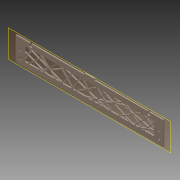
# Autodesk Inventor part: Panel_front
Saved by Autodesk Inventor 2013 (Build 170138000, 138)
## iProperties
Created: 2013-02-02
Part Number: Panel_front
Material: Aluminum 6061
Document SubType Name: Modeling
Designer: xylzlyx
Density: 1 g/cm^3
Author: xylzlyx
Autodesk Inventor part; units mm, degrees
ref_plane "YZ Plane" through (0, 0, 0) normal (1, 0, 0) x (0, 1, 0)
ref_plane "XZ Plane" through (0, 0, 0) normal (0, 1, 0) x (-1, 0, 0)
ref_plane "XY Plane" through (0, 0, 0) normal (0, 0, 1) x (1, 0, 0)
ref_plane "Work Plane1" through (0, 0, -9.525) normal (0, 0, 1) x (1, 0, 0)
sketch "Sketch1" plane through (0, 0, -9.525) normal (0, 0, 1) x (1, 0, 0)
  line L0 (381, -60.8043) -> (381, -64.0283) construction
  line L1 (381, -64.0283) -> (0, -64.0283) construction
  line L2 (0, -64.0283) -> (0, -60.8043) construction
  line L3 (0, -60.8043) -> (381, -60.8043) construction
  line L4 (381, 0) -> (0, 0) construction
  line L5 (0, 0) -> (0, 3.175) construction
  line L6 (0, 3.175) -> (381, 3.175) construction
  line L7 (381, 3.175) -> (381, 0) construction
  line L8 (381, -60.8043) -> (0, -60.8043)
  line L9 (0, -60.8043) -> (0, 0)
  line L10 (0, 0) -> (381, 0)
  line L11 (381, 0) -> (381, -60.8043)
  constraints: 24 end point, 5 horizontal, 4 coincident, 4 vertical, 2 parallel, 1 perpendicular, 8 other
extrude "FrontPanel" add sketch "Sketch1" against normal blind 3.175
fillet "CornerFillet" radius 1 4 edges at (381, -60.8043, -11.1125) (0, -60.8043, -11.1125) (0, 0, -11.1125) (381, 0, -11.1125)
sketch "ScrewSlotSketch" plane through (0, 0, -9.525) normal (0, 0, 1) x (1, 0, 0)
  line L0 (368.3, -28.0035) -> (368.3, -1) projected
  line L1 (12.7, -1) -> (12.7, -28.0035) projected
  line L2 (381, 0) -> (0, 0) construction
  line L3 (0, 0) -> (0, 3.175) construction
  line L4 (0, 3.175) -> (381, 3.175) construction
  line L5 (381, 3.175) -> (381, 0) construction
  line L6 (381, -60.8043) -> (381, -64.0283) construction
  line L7 (381, -64.0283) -> (0, -64.0283) construction
  line L8 (0, -64.0283) -> (0, -60.8043) construction
  line L9 (0, -60.8043) -> (381, -60.8043) construction
  line L10 (344.7987, -8.89) -> (344.7987, 3.175)
  line L11 (344.7987, 3.175) -> (341.0014, 3.175)
  line L12 (341.0014, 3.175) -> (341.0014, -8.89)
  line L13 (341.0014, -8.89) -> (344.7987, -8.89)
  line L14 (346.9958, -8.89) -> (338.8043, -8.89)
  line L15 (338.8043, -8.89) -> (338.8043, -5.8579)
  line L16 (338.8043, -5.8579) -> (346.9958, -5.8579)
  line L17 (346.9958, -5.8579) -> (346.9958, -8.89)
  line L18 (36.2014, -8.89) -> (39.9987, -8.89)
  line L19 (39.9987, -8.89) -> (39.9987, 3.175)
  line L20 (39.9987, 3.175) -> (36.2014, 3.175)
  line L21 (36.2014, 3.175) -> (36.2014, -8.89)
  line L22 (34.0043, -8.89) -> (42.1958, -8.89)
  line L23 (42.1958, -8.89) -> (42.1958, -5.8579)
  line L24 (42.1958, -5.8579) -> (34.0043, -5.8579)
  line L25 (34.0043, -5.8579) -> (34.0043, -8.89)
  point P0 (342.9, 3.175)
  point P1 (342.9, -8.89)
  point P2 (38.1, -8.89)
  point P3 (38.1, 3.175)
  dimension "d4" = 12.065
  dimension "d6" = 3.7973
  dimension "d7" = 25.4
  dimension "d8" = 8.1915
  dimension "d9" = 3.0321
  dimension "d10" = 3.7973
  dimension "d11" = 12.065
  dimension "d12" = 8.1915
  dimension "d13" = 3.0321
  dimension "d14" = 25.4
  constraints: 48 end point, 11 parallel, 6 horizontal, 6 midpoint, 4 vertical, 2 perpendicular, 2 point on line, 1 collinear, 7 other
  measures "d4" distance of L10.start L10.end
  measures "d6" distance of L10.end L11.end
  measures "d7" distance from line of L0 point (342.9, 3.175)
  measures "d8" distance of L14.start L14.end
  measures "d9" distance of L14.end L15.end
  measures "d10" distance of L19.end L20.end
  measures "d11" distance of L20.end L18.start
  measures "d12" distance of L22.start L22.end
  measures "d13" distance of L22.end L23.end
  measures "d14" distance from line of L1 point (38.1, 3.175)
extrude "ScrewSlotExtrusion" cut sketch "ScrewSlotSketch" against normal blind 3.175
fillet "ScrewSlotFillet" radius 0.5 16 edges at (344.7987, 0, -11.1125) (341.0014, 0, -11.1125) (344.7987, -5.8579, -11.1125) (341.0014, -5.8579, -11.1125) (338.8043, -5.8579, -11.1125) (338.8043, -8.89, -11.1125) (346.9958, -8.89, -11.1125) (346.9958, -5.8579, -11.1125) (42.1958, -8.89, -11.1125) (42.1958, -5.8579, -11.1125) (39.9987, -5.8579, -11.1125) (39.9987, 0, -11.1125) (36.2014, 0, -11.1125) (36.2014, -5.8579, -11.1125) (34.0043, -5.8579, -11.1125) (34.0043, -8.89, -11.1125)
sketch "ScrewHoleSketch" plane through (0, 0, -9.525) normal (0, 0, 1) x (1, 0, 0)
  line L0 (34.0043, -8.39) -> (34.0043, -6.3579) projected
  line L1 (368.3, -28.5035) -> (371.475, -28.5035) projected
  line L2 (371.475, -32.3008) -> (368.3, -32.3008) projected
  line L3 (9.525, -28.5035) -> (12.7, -28.5035) projected
  line L4 (12.7, -32.3008) -> (9.525, -32.3008) projected
  line L5 (371.475, -28.5035) -> (371.475, -32.3008) construction
  line L6 (9.525, -28.5035) -> (9.525, -32.3008) construction
  point P0 (0, 0)
  point P1 (11.1125, -30.4021)
  point P2 (369.8875, -30.4021)
  point P3 (369.8875, -28.5035)
  point P4 (371.475, -30.4021)
  point P5 (9.525, -30.4021)
  point P6 (11.1125, -28.5035)
  constraints: 4 end point, 4 midpoint, 2 horizontal alignment, 2 parallel, 2 vertical alignment
hole "ScrewHoles" at (11.1125, -30.4021, -9.525) at (369.8875, -30.4021, -9.525) direction (0, 0, -1) diameter 3.7973 end through all
sketch "BottomTabSketch" plane through (40.4987, 0, -9.525) normal (0, 1, 0) x (1, 0, 0)
  line L0 (162.7014, 3.175) -> (137.3014, 3.175)
  line L1 (137.3014, 3.175) -> (137.3014, 0)
  line L2 (137.3014, 0) -> (162.7014, 0)
  line L3 (162.7014, 0) -> (162.7014, 3.175)
  line L4 (137.0473, 2.929) -> (137.0473, 0.246) projected
  line L5 (137.5473, -0.254) -> (162.4553, -0.254) projected
  point P0 (0, 3.175)
  point P1 (-40.4987, -9.525)
  point P2 (137.3014, 1.5875)
  point P3 (137.0473, 1.5875)
  point P4 (150.0014, 0)
  point P5 (150.0013, -0.254)
  dimension "d29" = 25.4
  constraints: 8 end point, 4 midpoint, 2 horizontal alignment, 2 parallel, 1 horizontal, 1 perpendicular, 1 vertical alignment
  measures "d29" distance of L0.start L0.end
extrude "BottomTab" add sketch "BottomTabSketch" along normal blind 3.175
fillet "BottomTabFillet" radius 0.5 4 edges at (177.8, 0, -11.1125) (177.8, 3.175, -11.1125) (203.2, 3.175, -11.1125) (203.2, 0, -11.1125)
sketch "SlotSketch" plane through (0, 0, -9.525) normal (0, 0, 1) x (1, 0, 0)
  circle A0 centre (11.1125, -30.4021) radius 1.8986 projected
  circle A1 centre (369.8875, -30.4021) radius 1.8986 projected
  line L0 (371.729, -50.6197) -> (368.046, -50.6197)
  line L1 (368.046, -50.6197) -> (368.046, -40.5867)
  line L2 (368.046, -40.5867) -> (371.729, -40.5867)
  line L3 (371.729, -40.5867) -> (371.729, -50.6197)
  line L4 (12.954, -50.6197) -> (9.271, -50.6197)
  line L5 (9.271, -50.6197) -> (9.271, -40.5867)
  line L6 (9.271, -40.5867) -> (12.954, -40.5867)
  line L7 (12.954, -40.5867) -> (12.954, -50.6197)
  line L8 (380, -60.8043) -> (1, -60.8043) projected
  line L9 (203.2, 0.5) -> (203.2, 2.675) projected
  line L10 (11.1125, -30.4021) -> (11.1125, -60.8043) construction
  line L11 (369.8875, -30.4021) -> (369.8875, -60.8043) construction
  point P0 (0, 0)
  point P1 (12.954, -45.6032)
  point P2 (11.1125, -45.6032)
  point P3 (11.1125, -50.6197)
  point P4 (369.8875, -45.6032)
  point P5 (371.729, -45.6032)
  point P6 (369.8875, -50.6197)
  dimension "d34" = 10.033
  dimension "d36" = 3.683
  dimension "d37" = 10.033
  dimension "d38" = 3.683
  constraints: 20 end point, 6 midpoint, 6 parallel, 2 horizontal, 2 horizontal alignment, 2 perpendicular, 2 point on line, 2 vertical alignment
  measures "d34" distance of L0.end L1.end
  measures "d36" distance of L0.start L0.end
  measures "d37" distance of L6.end L4.start
  measures "d38" distance of L4.start L4.end
extrude "Extrusion4" cut sketch "SlotSketch" against normal blind 3.175 contours L0 L1 L2 L3 | L4 L5 L6 L7
fillet "Fillet5" radius 0.5 8 edges at (368.046, -40.5867, -11.1125) (371.729, -40.5867, -11.1125) (371.729, -50.6197, -11.1125) (368.046, -50.6197, -11.1125) (9.271, -40.5867, -11.1125) (12.954, -40.5867, -11.1125) (12.954, -50.6197, -11.1125) (9.271, -50.6197, -11.1125)
sketch "Sketch6" plane through (0, 0, -9.525) normal (0, 0, 1) x (1, 0, 0)
  line L0 (380, -60.8043) -> (1, -60.8043) projected
  line L1 (203.7, 0) -> (340.5014, 0) projected
  circle A0 centre (11.1125, -30.4021) radius 1.8986 projected
  circle A1 centre (369.8875, -30.4021) radius 1.8986 projected
  line L2 (357.1875, -48.1043) -> (23.8125, -48.1043)
  line L3 (23.8125, -48.1043) -> (23.8125, -12.7)
  line L4 (23.8125, -12.7) -> (357.1875, -12.7)
  line L5 (357.1875, -12.7) -> (357.1875, -48.1043)
  point P0 (0, 0)
  dimension "d42" = 12.7
  dimension "d43" = 12.7
  dimension "d44" = 12.7
  dimension "d45" = 12.7
  constraints: 8 end point, 2 parallel, 1 horizontal, 1 perpendicular
  measures "d42" distance from line of L0 L2.start
  measures "d43" distance between parallel lines of L1 L4
  measures "d44" distance from line of A1.centre L5
  measures "d45" distance from line of A0.centre L3
extrude "Extrusion5" cut sketch "Sketch6" against normal blind 25.4 contours L2 L3 L4 L5
fillet "Fillet6" radius 0.5 4 edges at (357.1875, -48.1043, -11.1125) (357.1875, -12.7, -11.1125) (23.8125, -48.1043, -11.1125) (23.8125, -12.7, -11.1125)
sketch "Sketch7" plane through (0, 0, -9.525) normal (0, 0, 1) x (1, 0, 0)
  line L0 (357.1875, -13.2) -> (357.1875, -47.6043) projected
  line L1 (356.6875, -48.1043) -> (24.3125, -48.1043) projected
  line L2 (23.8125, -47.6043) -> (23.8125, -13.2) projected
  line L3 (24.3125, -12.7) -> (356.6875, -12.7) projected
  arc A0 (357.1875, -13.2) -> (356.6875, -12.7) centre (356.6875, -13.2) ccw projected
  line L4 (203.7, 0) -> (340.5014, 0) projected
  line L5 (357.1875, -36.7105) -> (321.9415, -48.1043)
  line L6 (357.1875, -21.5969) -> (332.397, -48.1043)
  line L7 (344.6458, -12.7) -> (309.178, -48.1043)
  line L8 (326.9119, -12.7) -> (268.5984, -48.1043)
  line L9 (304.4629, -12.7) -> (185.3162, -48.1043)
  line L10 (278.4902, -12.7) -> (215.3456, -48.1043)
  line L11 (237.5513, -12.7) -> (203.2, -48.1043)
  line L12 (212.9458, -12.7) -> (157.4642, -48.1043)
  line L13 (168.7522, -12.7) -> (144.5905, -48.1043)
  line L14 (147.217, -12.7) -> (120.8379, -48.1043)
  line L15 (131.8636, -12.7) -> (62.8918, -48.1043)
  line L16 (105.8433, -12.7) -> (72.2367, -48.1043)
  line L17 (74.5284, -12.7) -> (34.5043, -48.1043)
  line L18 (41.1958, -12.7) -> (23.8125, -42.1574)
  line L19 (357.1875, -36.7105) -> (357.1875, -34.575)
  line L20 (357.1875, -34.575) -> (315.3354, -48.1043)
  line L21 (321.9415, -48.1043) -> (315.3354, -48.1043)
  line L22 (357.1875, -21.5969) -> (357.1875, -18.622)
  line L23 (357.1875, -18.622) -> (329.6149, -48.1043)
  line L24 (329.6149, -48.1043) -> (332.397, -48.1043)
  line L25 (344.6458, -12.7) -> (341.7696, -12.7)
  line L26 (341.7696, -12.7) -> (306.3017, -48.1043)
  line L27 (309.178, -48.1043) -> (306.3017, -48.1043)
  line L28 (326.9119, -12.7) -> (322.9965, -12.7)
  line L29 (322.9965, -12.7) -> (264.683, -48.1043)
  line L30 (264.683, -48.1043) -> (268.5984, -48.1043)
  line L31 (304.4629, -12.7) -> (297.3291, -12.7)
  line L32 (297.3291, -12.7) -> (178.1824, -48.1043)
  line L33 (185.3162, -48.1043) -> (178.1824, -48.1043)
  line L34 (278.4902, -12.7) -> (274.3353, -12.7)
  line L35 (274.3353, -12.7) -> (211.1907, -48.1043)
  line L36 (208.3319, -48.1043) -> (215.3456, -48.1043)
  line L37 (237.5513, -12.7) -> (234.72, -12.7)
  line L38 (234.72, -12.7) -> (200.3687, -48.1043)
  line L39 (203.2, -48.1043) -> (200.3687, -48.1043)
  line L40 (212.9458, -12.7) -> (209.1683, -12.7)
  line L41 (209.1683, -12.7) -> (153.6867, -48.1043)
  line L42 (157.4642, -48.1043) -> (153.6867, -48.1043)
  line L43 (168.7522, -12.7) -> (166.2921, -12.7)
  line L44 (166.2921, -12.7) -> (142.1304, -48.1043)
  line L45 (142.1304, -48.1043) -> (144.5905, -48.1043)
  line L46 (147.217, -12.7) -> (144.683, -12.7)
  line L47 (144.683, -12.7) -> (118.3039, -48.1043)
  line L48 (120.8379, -48.1043) -> (118.3039, -48.1043)
  line L49 (131.8636, -12.7) -> (127.4139, -12.7)
  line L50 (127.4139, -12.7) -> (58.4422, -48.1043)
  line L51 (58.4422, -48.1043) -> (62.8918, -48.1043)
  line L52 (105.8433, -12.7) -> (103.0416, -12.7)
  line L53 (103.0416, -12.7) -> (69.4351, -48.1043)
  line L54 (69.4351, -48.1043) -> (72.2367, -48.1043)
  line L55 (74.5284, -12.7) -> (71.4615, -12.7)
  line L56 (71.4615, -12.7) -> (31.4373, -48.1043)
  line L57 (34.5043, -48.1043) -> (31.4373, -48.1043)
  line L58 (41.1958, -12.7) -> (38.8363, -12.7)
  line L59 (38.8363, -12.7) -> (23.8125, -38.1592)
  line L60 (23.8125, -42.1574) -> (23.8125, -38.1592)
  point P0 (0, 0)
  dimension "d49" = 23.5105
  dimension "d50" = 8.3969
  dimension "d51" = 72.086
  dimension "d52" = 43.083
  dimension "d53" = 12.0417
  dimension "d54" = 29.7756
  dimension "d55" = 135.051
  dimension "d56" = 148.736
  dimension "d57" = 52.2246
  dimension "d58" = 163.451
  dimension "d59" = 78.1973
  dimension "d60" = 150.721
  dimension "d61" = 119.1362
  dimension "d62" = 134.135
  dimension "d63" = 143.7417
  dimension "d64" = 147.457
  dimension "d65" = 187.9353
  dimension "d66" = 124.312
  dimension "d67" = 209.4705
  dimension "d68" = 126.689
  dimension "d69" = 224.8239
  dimension "d70" = 152.828
  dimension "d71" = 250.8442
  dimension "d72" = 133.508
  dimension "d73" = 282.1591
  dimension "d74" = 138.505
  dimension "d75" = 315.4918
  dimension "d76" = 120.545
  dimension "d77" = 2.032
  dimension "d78" = 2.032
  dimension "d79" = 2.032
  dimension "d80" = 2.032
  dimension "d81" = 2.032
  dimension "d82" = 2.032
  dimension "d83" = 2.032
  dimension "d84" = 2.032
  dimension "d85" = 2.032
  dimension "d86" = 2.032
  dimension "d87" = 2.032
  dimension "d88" = 2.032
  dimension "d89" = 2.032
  dimension "d90" = 2.032
  constraints: 112 end point, 16 parallel, 10 horizontal, 6 point on line, 1 collinear, 53 other
  measures "d49" vertical distance of A0.centre L5.start
  measures "d50" vertical distance of A0.centre L6.start
  measures "d51" angle of L0 L5
  measures "d52" angle of L0 L6
  measures "d53" distance of A0.end L7.start
  measures "d54" distance of A0.end L8.start
  measures "d55" angle to the sketch x axis of L7
  measures "d56" angle to the sketch x axis of L8
  measures "d57" distance of A0.end L9.start
  measures "d58" angle to the sketch x axis of L9
  measures "d59" distance of A0.end L10.start
  measures "d60" angle to the sketch x axis of L10
  measures "d61" distance of A0.end L11.start
  measures "d62" angle to the sketch x axis of L11
  measures "d63" distance of A0.end L12.start
  measures "d64" angle to the sketch x axis of L12
  measures "d65" distance of A0.end L13.start
  measures "d66" angle to the sketch x axis of L13
  measures "d67" distance of A0.end L14.start
  measures "d68" angle to the sketch x axis of L14
  measures "d69" distance of A0.end L15.start
  measures "d70" angle to the sketch x axis of L15
  measures "d71" distance of A0.end L16.start
  measures "d72" angle to the sketch x axis of L16
  measures "d73" distance of A0.centre L17.start
  measures "d74" angle to the sketch x axis of L17
  measures "d75" distance of A0.centre L18.start
  measures "d76" angle to the sketch x axis of L18
  measures "d77" distance between parallel lines of L5 L20
  measures "d78" distance between parallel lines of L6 L23
  measures "d79" distance between parallel lines of L7 L26
  measures "d80" distance between parallel lines of L8 L29
  measures "d81" distance between parallel lines of L9 L32
  measures "d82" distance between parallel lines of L10 L35
  measures "d83" distance between parallel lines of L38 L11
  measures "d84" distance between parallel lines of L41 L12
  measures "d85" distance between parallel lines of L44 L13
  measures "d86" distance between parallel lines of L14 L47
  measures "d87" distance between parallel lines of L15 L50
  measures "d88" distance between parallel lines of L16 L53
  measures "d89" distance between parallel lines of L17 L56
  measures "d90" distance between parallel lines of L18 L59
extrude "Hash1" add sketch "Sketch7" against normal blind 3.175 contours L0 L6 L20 L23 | L23 L5 L1 L20 | L20 L6 L5 L23 | L7 L1 L26 L3 | L0 L5 L6 L20 | L5 L6 L1 L23 | L8 L1 L29 L3 | L9 L10 L32 L3 | L10 L1 L35 L9 | L9 L35 L32 L10 | L10 L32 L35 L3 | L9 L11 L32 L35 | L11 L1 L38 L9 | L9 L38 L32 L11 | L11 L32 L38 L3 | L9 L1 L32 L38 | L12 L1 L41 L3 | L13 L1 L44 L3 | L14 L1 L47 L3 | L15 L16 L50 L3 | L16 L1 L53 L15 | L15 L53 L50 L16 | L16 L50 L53 L3 | L15 L1 L50 L53 | L17 L1 L56 L3 | L2 L59 L3 L18
sketch "Sketch8" plane through (0, 0, -9.525) normal (0, 0, 1) x (1, 0, 0)
  line L0 (212.9458, -12.7) -> (234.72, -12.7) projected
  line L1 (304.4629, -12.7) -> (322.9965, -12.7) projected
  line L2 (264.683, -48.1043) -> (215.3456, -48.1043) projected
  line L3 (200.3687, -48.1043) -> (185.3162, -48.1043) projected
  line L4 (237.5513, -12.7) -> (274.3353, -12.7) projected
  line L5 (118.3039, -48.1043) -> (72.2367, -48.1043) projected
  line L6 (74.5284, -12.7) -> (103.0416, -12.7) projected
  line L7 (357.1875, -36.7105) -> (357.1875, -47.6043) projected
  arc A0 (357.1875, -13.2) -> (356.6875, -12.7) centre (356.6875, -13.2) ccw projected
  line L8 (329.6149, -48.1043) -> (321.9415, -48.1043) projected
  line L9 (153.6867, -48.1043) -> (144.5905, -48.1043) projected
  line L10 (168.7522, -12.7) -> (209.1683, -12.7) projected
  line L11 (306.3017, -48.1043) -> (268.5984, -48.1043) projected
  line L12 (326.9119, -12.7) -> (341.7696, -12.7) projected
  line L13 (147.217, -12.7) -> (166.2921, -12.7) projected
  line L14 (23.8125, -38.1592) -> (23.8125, -13.2) projected
  line L15 (24.3125, -12.7) -> (38.8363, -12.7) projected
  line L16 (105.8433, -12.7) -> (127.4139, -12.7) projected
  line L17 (41.1958, -12.7) -> (71.4615, -12.7) projected
  line L18 (278.4902, -12.7) -> (297.3291, -12.7) projected
  line L19 (357.1875, -21.5969) -> (357.1875, -34.575) projected
  line L20 (243.5183, -12.7) -> (357.1875, -39.9851)
  line L21 (279.4501, -12.7) -> (324.0356, -48.1043)
  line L22 (206.4666, -12.7) -> (243.5183, -48.1043)
  line L23 (171.4741, -12.7) -> (198.865, -48.1043)
  line L24 (120.8379, -12.7) -> (227.4264, -48.1043)
  line L25 (112.4755, -12.7) -> (146.4133, -48.1043)
  line L26 (328.1908, -12.7) -> (357.1875, -33.5005)
  line L27 (219.5665, -12.7) -> (293.0889, -48.1043)
  line L28 (60.7242, -12.7) -> (101.1114, -48.1043)
  line L29 (29.3613, -12.7) -> (116.1142, -48.1043)
  line L30 (23.8125, -28.5035) -> (75.6529, -48.1043)
  line L31 (328.1908, -12.7) -> (331.677, -12.7)
  line L32 (331.677, -12.7) -> (357.1875, -30.9997)
  line L33 (357.1875, -33.5005) -> (357.1875, -30.9997)
  line L34 (279.4501, -12.7) -> (282.7177, -12.7)
  line L35 (282.7177, -12.7) -> (327.3032, -48.1043)
  line L36 (327.3032, -48.1043) -> (324.0356, -48.1043)
  line L37 (243.5183, -12.7) -> (252.224, -12.7)
  line L38 (252.224, -12.7) -> (357.1875, -37.8954)
  line L39 (357.1875, -37.8954) -> (357.1875, -39.9851)
  line L40 (219.5665, -12.7) -> (224.25, -12.7)
  line L41 (224.25, -12.7) -> (297.7725, -48.1043)
  line L42 (297.7725, -48.1043) -> (293.0889, -48.1043)
  line L43 (243.5183, -48.1043) -> (246.4596, -48.1043)
  line L44 (246.4596, -48.1043) -> (209.4079, -12.7)
  line L45 (209.4079, -12.7) -> (206.4666, -12.7)
  line L46 (227.4264, -48.1043) -> (233.8726, -48.1043)
  line L47 (233.8726, -48.1043) -> (127.2841, -12.7)
  line L48 (120.8379, -12.7) -> (127.2841, -12.7)
  line L49 (146.4133, -48.1043) -> (149.2281, -48.1043)
  line L50 (149.2281, -48.1043) -> (115.2903, -12.7)
  line L51 (115.2903, -12.7) -> (112.4755, -12.7)
  line L52 (116.1142, -48.1043) -> (121.492, -48.1043)
  line L53 (121.492, -48.1043) -> (34.7391, -12.7)
  line L54 (34.7391, -12.7) -> (29.3613, -12.7)
  line L55 (60.7242, -12.7) -> (63.8068, -12.7)
  line L56 (63.8068, -12.7) -> (104.194, -48.1043)
  line L57 (101.1114, -48.1043) -> (104.194, -48.1043)
  line L58 (75.6529, -48.1043) -> (81.3985, -48.1043)
  line L59 (81.3985, -48.1043) -> (23.8125, -26.3311)
  line L60 (23.8125, -26.3311) -> (23.8125, -28.5035)
  line L61 (198.865, -48.1043) -> (201.4341, -48.1043)
  line L62 (201.4341, -48.1043) -> (174.0432, -12.7)
  line L63 (174.0432, -12.7) -> (171.4741, -12.7)
  point P0 (0, 0)
  dimension "d93" = 28.4967
  dimension "d94" = 77.2374
  dimension "d95" = 113.1692
  dimension "d96" = 137.121
  dimension "d97" = 150.2209
  dimension "d98" = 185.2134
  dimension "d99" = 235.8496
  dimension "d100" = 244.212
  dimension "d101" = 295.9633
  dimension "d102" = 327.3262
  dimension "d103" = 15.3035
  dimension "d104" = 144.347
  dimension "d105" = 141.548
  dimension "d106" = 166.502
  dimension "d107" = 154.287
  dimension "d108" = 136.302
  dimension "d109" = 127.728
  dimension "d110" = 161.626
  dimension "d111" = 133.788
  dimension "d112" = 138.762
  dimension "d113" = 157.799
  dimension "d114" = 69.288
  dimension "d115" = 2.032
  dimension "d116" = 2.032
  dimension "d117" = 2.032
  dimension "d118" = 2.032
  dimension "d119" = 2.032
  dimension "d120" = 2.032
  dimension "d121" = 2.032
  dimension "d122" = 2.032
  dimension "d123" = 2.032
  dimension "d124" = 2.032
  dimension "d125" = 2.032
  constraints: 88 end point, 45 point on line, 15 parallel, 8 collinear
  measures "d93" distance of A0.end L26.start
  measures "d94" distance of L21.start A0.end
  measures "d95" distance of A0.end L20.start
  measures "d96" distance of A0.end L27.start
  measures "d97" distance of A0.end L22.start
  measures "d98" distance of A0.end L23.start
  measures "d99" horizontal distance of L24.start A0.centre
  measures "d100" distance of A0.end L25.start
  measures "d101" distance of L28.start A0.end
  measures "d102" distance of A0.end L29.start
  measures "d103" distance of L14.end L30.start
  measures "d104" angle of L1 L26
  measures "d105" angle of L4 L21
  measures "d106" angle of L0 L20
  measures "d107" angle of L10 L27
  measures "d108" angle of L10 L22
  measures "d109" angle of L13 L23
  measures "d110" angle of L6 L24
  measures "d111" angle of L6 L25
  measures "d112" angle of L17 L28
  measures "d113" angle of L15 L29
  measures "d114" angle of L14 L30
  measures "d115" distance between parallel lines of L26 L32
  measures "d116" distance between parallel lines of L20 L38
  measures "d117" distance between parallel lines of L21 L35
  measures "d118" distance between parallel lines of L27 L41
  measures "d119" distance between parallel lines of L22 L44
  measures "d120" distance between parallel lines of L24 L47
  measures "d121" distance between parallel lines of L23 L62
  measures "d122" distance between parallel lines of L25 L50
  measures "d123" distance between parallel lines of L29 L53
  measures "d124" distance between parallel lines of L28 L56
  measures "d125" distance between parallel lines of L30 L59
extrude "Hash2" add sketch "Sketch8" against normal blind 3.175 contours L0 L41 L11 L27 | L2 L22 L10 L45 L44 | L2 L24 L62 L47 | L62 L24 L23 L47 | L47 L23 L10 L62 | L62 L61 L3 L23 L24 | L23 L24 L16 L47 | L4 L38 L21 L20 | L21 L38 L35 L20 | L20 L35 L8 L21 | L21 L18 L35 L38 | L35 L38 L7 L20 | L5 L29 L56 L53 L52 | L5 L28 L29 L56 | L29 L28 L53 L56 | L53 L28 L17 L56 | L29 L15 L53 L28 | L5 L30 L14 L59 | L9 L25 L16 L50 | L12 L32 L19 L26
equation "\"d4\" = ScrewLen"
equation "\"d6\" = ScrewHoleD"
equation "\"d7\" = ScrewHoleDist"
equation "\"d8\" = NutFlatsGap"
equation "\"d9\" = NutHeightGap"
equation "\"d10\" = ScrewHoleD"
equation "\"d11\" = ScrewLen"
equation "\"d12\" = NutFlatsGap"
equation "\"d13\" = NutHeightGap"
equation "\"d14\" = ScrewHoleDist"
equation "\"d21\" = SlotFilletRad"
equation "\"d22\" = ScrewHoleD"
equation "\"d29\" = TabLength"
equation "\"d33\" = SlotFilletRad"
equation "\"d34\" = SmallSlotLength"
equation "\"d36\" = SlotWidth"
equation "\"d37\" = SmallSlotLength"
equation "\"d38\" = SlotWidth"
equation "\"d41\" = SlotFilletRad"
equation "\"d42\" = EdgeThickness"
equation "\"d43\" = EdgeThickness"
equation "\"d44\" = EdgeThickness"
equation "\"d45\" = EdgeThickness"
equation "\"d48\" = SlotFilletRad"
equation "\"ScrewLen\" = 12.065"
equation "\"ScrewHoleD\" = 3.7973"
equation "\"NutFlatsGap\" = 8.1915"
equation "\"NutHeightGap\" = 3.032125"
equation "\"SlotFilletRad\" = 0.5"
equation "\"TabLength\" = 25.4"
equation "\"SmallSlotLength\" = 10.033"
equation "\"SlotWidth\" = 3.683"
equation "\"EdgeThickness\" = 12.7"
equation "\"ScrewHoleDist\" = 25.4"
body "Solid1"
